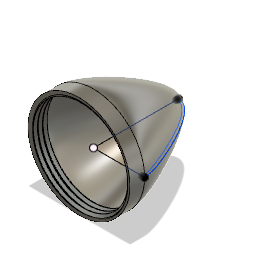
FalconHeavy-BoosterCone (Autodesk Fusion 360 design; units mm, degrees)
Autodesk Fusion 360 part; units mm, degrees
sketch "Sketch1" plane through (0, 0, 0) normal (0, 1, 0) x (1, 0, 0)
  line L0 (0, 0) -> (21, 0)
  line L1 (21, 0) -> (20.2, 0)
  line L2 (0, 0) -> (0, 30)
  line L3 (0, 30) -> (0, 29.2)
  spline S0 degree 5 poles (21, 0) (21, 1.069) (20.7385, 3.4242) (19.5623, 7.608) (16.6561, 14.1612) (11.6344, 22.3909) (7.0757, 27.4589) (3.5573, 29.5377) (1.1895, 30) (0, 30) knots 0 0 0 0 0 0 0.2 0.4 0.6 0.8 1 1 1 1 1 1
  line L4 (2.5, 30) -> (-2.5, 30)
  line L5 (21, -2.5) -> (21, 2.5)
  spline S1 degree 5 poles (20.2, 0) (20.2156, 0.8446) (19.9823, 2.8161) (18.8396, 6.619) (15.969, 12.993) (11.0272, 21.3116) (6.6161, 26.5285) (3.29, 28.6915) (1.0932, 29.1882) (0, 29.2) knots 0 0 0 0 0 0 0.2 0.4 0.6 0.8 1 1 1 1 1 1
  line L6 (2.3018, 29.1752) -> (-2.3018, 29.2248)
  line L7 (20.1637, -1.9685) -> (20.2363, 1.9685)
  line L8 (21, 0) -> (21, -6)
  line L9 (20.2, 0) -> (20.2, -6)
  line L10 (21, -6) -> (20.2, -6)
  dimension "d1" = 21
  dimension "d3" = 0.8
  dimension "d4" = 30
  dimension "d5" = 0.8
  dimension "d6" = 6
  dimension "d7" = 6
  dimension "d8" = 0.8
  constraint coincident L0.start L2.start
  constraint horizontal L0
  constraint parallel L0 L1
  constraint vertical L2
  constraint parallel L2 L3
  constraint midpoint L2.end L4
  constraint midpoint L0.end L5
  constraint midpoint L3.end L6
  constraint midpoint L1.end L7
  constraint perpendicular L0 L8
  constraint perpendicular L1 L9
  constraint perpendicular L9 L10
  measures "d1" distance of L0.start L0.end
  measures "d3" distance of L0.end L1.end
  measures "d4" distance of L0.start L2.end
  measures "d5" distance of L2.end L3.end
  measures "d6" distance of L0.end L8.end
  measures "d7" distance of L1.end L9.end
  measures "d8" distance of L8.end L9.end
revolve "Revolve1" add sketch "Sketch1" angle 360 about axis through (0, 0, 0) along (0, 0, -1) contours L0 L1 L5 L8 L9 L10
thread "Thread1" "ISO Metric profile 40.0 M40x2 6H" major diameter 40.2565 minor diameter 38.0224 pitch 2 angle 60 modelled right hand crest width 0.25 on face at (20.1749, 1.0069, 2) crest through (19.0112, 0, -1.125)
sketch "Sketch2" plane through (0, 0, 0) normal (0, 1, 0) x (1, 0, 0)
  line L0 (0, 0) -> (0, 35)
  line L1 (0, 0) -> (21, 0)
  line L2 (21, 0) -> (20.2, 0)
  line L3 (0, 35) -> (0, 34.2)
  spline S0 degree 5 poles (21, 0) (21, 0.8402) (20.7151, 2.9246) (19.434, 7.2616) (16.2864, 14.9333) (10.9865, 25.2164) (6.417, 31.7208) (3.1206, 34.4035) (1.0234, 35) (0, 35) knots 0 0 0 0 0 0 0.2 0.4 0.6 0.8 1 1 1 1 1 1
  line L4 (2.1, 35) -> (-2.1, 35)
  line L5 (21, -2) -> (21, 2)
  spline S1 degree 5 poles (20.2, 0) (20.2108, 0.565) (19.9557, 2.182) (18.7435, 6.0668) (15.7279, 13.5544) (10.6266, 24.002) (6.2161, 30.7288) (3.0265, 33.5353) (0.9933, 34.1826) (0, 34.2) knots 0 0 0 0 0 0 0.2 0.4 0.6 0.8 1 1 1 1 1 1
  line L6 (2.0456, 34.1641) -> (-2.0456, 34.2359)
  line L7 (20.1743, -1.341) -> (20.2257, 1.341)
  line L8 (0, 0) -> (21, 0)
  line L9 (0, 0) -> (0, 35)
  spline S2 degree 5 poles (21, 0) (21, 0.8402) (20.7151, 2.9246) (19.434, 7.2616) (16.2864, 14.9333) (10.9865, 25.2164) (6.417, 31.7208) (3.1206, 34.4035) (1.0234, 35) (0, 35) knots 0 0 0 0 0 0 0.2 0.4 0.6 0.8 1 1 1 1 1 1
  line L10 (21, -2) -> (21, 2)
  line L11 (2.1, 35) -> (-2.1, 35)
  line L12 (21, 0) -> (20.2, 0)
  spline S3 degree 5 poles (20.2, 0) (20.2108, 0.565) (19.9557, 2.182) (18.7435, 6.0668) (15.7279, 13.5544) (10.6266, 24.002) (6.2161, 30.7288) (3.0265, 33.5353) (0.9933, 34.1826) (0, 34.2) knots 0 0 0 0 0 0 0.2 0.4 0.6 0.8 1 1 1 1 1 1
  line L13 (20.1743, -1.341) -> (20.2257, 1.341)
  line L14 (2.0456, 34.1641) -> (-2.0456, 34.2359)
  line L15 (0, 35) -> (0, 34.2)
  dimension "d11" = 35
  dimension "d12" = 21
  dimension "d13" = 0.8
  dimension "d14" = 0.8
  dimension "d16" = 35
  dimension "d17" = 21
  dimension "d18" = 0.8
  dimension "d19" = 0.8
  constraint coincident L0.start L1.start
  constraint vertical L0
  constraint perpendicular L0 L1
  constraint parallel L1 L2
  constraint parallel L0 L3
  constraint midpoint L0.end L4
  constraint midpoint L1.end L5
  constraint midpoint L3.end L6
  constraint midpoint L2.end L7
  constraint vertical L9
  constraint perpendicular L8 L9
  constraint parallel L8 L12
  constraint parallel L9 L15
  constraint midpoint L0.end L11
  constraint midpoint L1.end L10
  constraint midpoint L3.end L14
  constraint midpoint L2.end L13
  measures "d11" distance of L0.start L0.end
  measures "d12" distance of L0.start L1.end
  measures "d13" distance of L1.end L2.end
  measures "d14" distance of L0.end L3.end
  measures "d16" distance of L0.start L0.end
  measures "d17" distance of L1.end L0.start
  measures "d18" distance of L1.end L2.end
  measures "d19" distance of L3.end L0.end
revolve "Revolve2" add sketch "Sketch2" angle 360 about axis through (0, 0, 0) along (0, 0, -1) contours L0 L1 L2 L3 S0 S1 L8 L9 S2 L12 S3 L15
equation "Wall_Thickness = 0.8 mm"
equation "d3 = Wall_Thickness"
equation "d5 = Wall_Thickness"
equation "d8 = Wall_Thickness"
equation "d13 = Wall_Thickness"
equation "d14 = Wall_Thickness"
equation "d18 = Wall_Thickness"
equation "d19 = Wall_Thickness"
